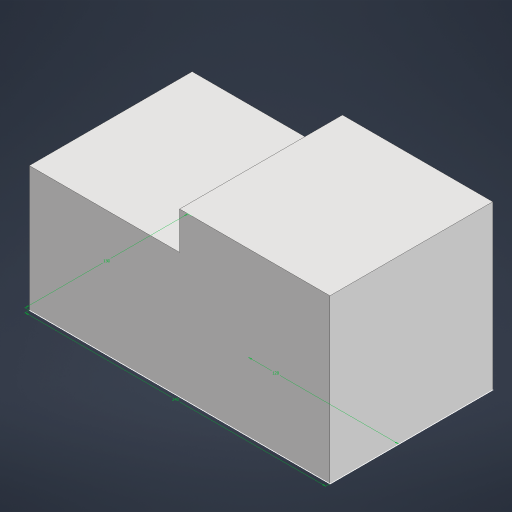
# Autodesk Inventor part: HotPlate
Saved by Autodesk Inventor 2024.2 (Build 282272000, 272)
## iProperties
Created: 2024-10-04
Part Number: HotPlate
Material: Generic
Document SubType Name: Modeling
Designer: jerem
Density: 1 g/cm^3
Appearance: Default
Author: jerem
Autodesk Inventor part; units mm, degrees
ref_plane "YZ Plane" through (0, 0, 0) normal (1, 0, 0) x (0, 1, 0)
ref_plane "XZ Plane" through (0, 0, 0) normal (0, 1, 0) x (-1, 0, 0)
ref_plane "XY Plane" through (0, 0, 0) normal (0, 0, 1) x (1, 0, 0)
sketch "Sketch1" plane through (0, 0, 0) normal (0, 1, 0) x (-1, 0, 0)
  line L0 (-120, -65) -> (120, -65)
  line L1 (120, -65) -> (120, 65)
  line L2 (120, 65) -> (-120, 65)
  line L3 (-120, 65) -> (-120, -65)
  line L4 (-120, -65) -> (120, 65) construction
  line L5 (120, -65) -> (-120, 65) construction
  line L6 (0, 65) -> (0, -65)
  point P0 (0, 0)
  dimension "d0" = 240
  dimension "d1" = 130
  dimension "d4" = 120
  constraints: 14 end point, 4 midpoint, 2 parallel, 2 perpendicular, 1 horizontal
  measures "d0" distance of L2.end L1.end
  measures "d1" distance of L1.end L0.end
  measures "d4" distance between parallel lines of L6 L3
extrude "Extrusion1" add sketch "Sketch1" along normal blind 100
extrude "Extrusion2" add sketch "Sketch1" along normal blind 30 from surface at 100 contours L3 L2 L6 L0
body "Solid1"
